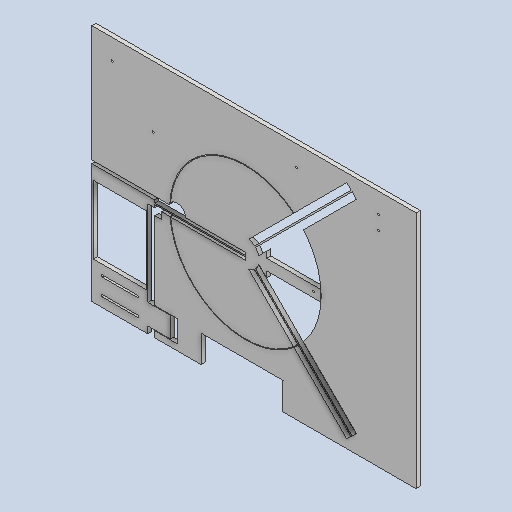
# Autodesk Inventor part: Wheel1
Saved by Autodesk Inventor 2023 (Build 270158000, 158)
## iProperties
Created: 2023-05-10
Part Number: Wheel1
Material: Generic
Document SubType Name: Modeling
Designer: Nathann
Density: 1 g/cm^3
Appearance: Default
Author: Nathann
Autodesk Inventor part; units mm, degrees
ref_plane "YZ Plane" through (0, 0, 0) normal (1, 0, 0) x (0, 1, 0)
ref_plane "XZ Plane" through (0, 0, 0) normal (0, 1, 0) x (-1, 0, 0)
ref_plane "XY Plane" through (0, 0, 0) normal (0, 0, 1) x (1, 0, 0)
sketch "Sketch1" plane through (0, 0, 0) normal (0, 0, 1) x (1, 0, 0)
  line L0 (0, 0) -> (-400, 0)
  line L1 (-400, 0) -> (-400, 350)
  line L2 (-400, 350) -> (0, 350)
  line L3 (0, 350) -> (0, 0)
  circle A0 centre (-175, 175) radius 110
  circle A1 centre (-175, 175) radius 20
  line L4 (-160.8579, 160.8579) -> (0, 0)
  line L5 (0, 350) -> (-160.8579, 189.1421)
  line L6 (-169.8236, 194.3185) -> (-26.5076, 337.6346)
  line L7 (-26.5076, 337.6346) -> (-12.3654, 323.4924)
  line L8 (-12.3654, 323.4924) -> (-155.6815, 180.1764)
  line L9 (-155.6815, 169.8236) -> (-12.1198, 26.262)
  line L10 (-169.8236, 155.6815) -> (-26.7532, 12.6111)
  line L11 (-26.7532, 12.6111) -> (-12.1198, 26.262)
  line L12 (-160.1684, 188.4173) -> (-18.7294, 329.8564)
  line L13 (-20.1436, 331.2706) -> (-161.5827, 189.8316)
  line L14 (-160.1684, 161.5827) -> (-18.7048, 20.1191)
  line L15 (-20.1682, 18.754) -> (-161.5827, 160.1684)
  circle A2 centre (-175, 175) radius 111
  line L16 (-400, 0) -> (-317.8714, 0)
  line L17 (-317.8714, 0) -> (-317.8714, 55)
  line L18 (-317.8714, 55) -> (-400, 55)
  line L19 (-400, 55) -> (-400, 0)
  line L20 (-317.8714, 0) -> (-307.8714, 0)
  line L21 (-307.8714, 0) -> (-307.8714, 155)
  line L22 (-317.8714, 155) -> (-317.8714, 0)
  line L23 (-317.8714, 55) -> (-320.1214, 55)
  line L24 (-320.1214, 55) -> (-320.1214, 155)
  line L25 (-320.1214, 155) -> (-317.8714, 155)
  line L26 (-317.8714, 155) -> (-317.8714, 55)
  line L27 (-400, 55) -> (-397.75, 55)
  line L28 (-397.75, 55) -> (-397.75, 155)
  line L29 (-397.75, 155) -> (-400, 155)
  line L30 (-400, 155) -> (-400, 55)
  line L31 (-400, 155) -> (-307.8714, 155)
  line L32 (-307.8714, 155) -> (-307.8714, 175)
  line L33 (-307.8714, 175) -> (-400, 175)
  line L34 (-400, 175) -> (-400, 155)
  line L35 (-175, 175) -> (-307.8714, 175)
  line L36 (-307.8714, 175) -> (-307.8714, 171)
  line L37 (-307.8714, 171) -> (-175, 171)
  line L38 (-175, 171) -> (-175, 175)
  line L39 (-307.8714, 169) -> (-175, 169)
  line L40 (-175, 169) -> (-175, 165)
  line L41 (-175, 165) -> (-307.8714, 165)
  line L42 (-307.8714, 165) -> (-307.8714, 169)
  line L43 (-317.8714, 155) -> (-297.8714, 155)
  line L44 (-297.8714, 155) -> (-297.8714, 165)
  line L45 (-297.8714, 165) -> (-317.8714, 165)
  line L46 (-317.8714, 165) -> (-317.8714, 155)
  line L47 (-400, 175) -> (-285.6082, 175)
  line L48 (-285.6082, 175) -> (-285.6082, 179.6746)
  line L49 (-285.6082, 179.6746) -> (-400, 179.6746)
  line L50 (-400, 179.6746) -> (-400, 175)
  line L51 (-317.8714, 40) -> (-285, 40)
  line L52 (-285, 40) -> (-285, 10)
  line L53 (-285, 10) -> (-317.8714, 10)
  line L54 (-317.8714, 10) -> (-317.8714, 40)
  line L55 (-307.8714, 53.2478) -> (-275, 53.2478)
  line L56 (-275, 53.2478) -> (-275, 41)
  line L57 (-275, 41) -> (-307.8714, 41)
  line L58 (-307.8714, 41) -> (-307.8714, 53.2478)
  line L59 (-275, 53.2478) -> (-257.3747, 53.2478)
  line L60 (-257.3747, 53.2478) -> (-257.3747, 0)
  line L61 (-257.3747, 0) -> (-275, 0)
  line L62 (-275, 0) -> (-275, 53.2478)
  line L63 (-275, 0) -> (-307.8714, 0)
  line L64 (-307.8714, 0) -> (-307.8714, 9)
  line L65 (-307.8714, 9) -> (-275, 9)
  line L66 (-275, 9) -> (-275, 0)
  point P0 (-19.4365, 330.5635)
  point P1 (-19.4365, 19.4365)
  point P2 (-89.7592, 246.0986)
  point P3 (-89.7592, 103.9014)
  point P4 (-90.4693, 104.6114)
  point P5 (-90.4693, 245.3886)
  point P6 (-104.6114, 259.5307)
  point P7 (-104.6114, 90.4693)
  point P8 (-103.9014, 89.7592)
  point P9 (-103.9014, 260.2408)
  point P10 (-317.8714, 27.5)
  point P11 (-285.5486, 165)
  point P12 (-284.5445, 165)
  point P13 (-317.8714, 0)
  point P14 (-285, 175)
  point P15 (-286, 175)
  point P16 (-285.8377, 169)
  point P17 (-194.0788, 169)
  point P18 (-192.3205, 165)
  point P19 (-97.9286, 96.5144)
  point P20 (-97.2214, 95.8072)
  point P21 (-284.8362, 169)
  point P22 (-96.5144, 97.9286)
  point P23 (-96.5144, 252.0714)
  point P24 (-97.9286, 253.4856)
  point P25 (-97.2214, 254.1928)
  point P26 (-95.8072, 252.7786)
  point P27 (-95.8072, 97.2214)
  point P28 (-285.9015, 179.6746)
  point P29 (-312.8714, 0)
  dimension "d7" = 40
  dimension "d0" = 350
  dimension "d1" = 400
  dimension "d4" = 175
  dimension "d5" = 175
  dimension "d6" = 220
  dimension "d8" = 10
  dimension "d9" = 10
  dimension "d10" = 10
  dimension "d11" = 10
  dimension "d12" = 1
  dimension "d13" = 1
  dimension "d14" = 1
  dimension "d15" = 1
  dimension "d16" = 200
  dimension "d17" = 200
  dimension "d18" = 222
  dimension "d19" = 100
  dimension "d20" = 2.25
  dimension "d21" = 2.25
  dimension "d22" = 10
  dimension "d24" = 20
  dimension "d25" = 0
  dimension "d26" = 6
  dimension "d27" = 4
  dimension "d28" = 4
  dimension "d29" = 20
  dimension "d30" = 0
  dimension "d31" = 1
  dimension "d32" = 1
  dimension "d33" = 10
  dimension "d34" = 30
  dimension "d35" = 10
  constraints: 134 end point, 33 parallel, 16 perpendicular, 15 point on line, 14 horizontal, 4 midpoint, 2 centre point, 2 coincident, 12 other
  measures "d0" distance of L2.end L0.start
  measures "d1" distance of L0.start L0.end
  measures "d4" distance from line of L3 A0.centre
  measures "d5" distance from line of L0 A0.centre
  measures "d6" diameter of A0
  measures "d8" distance between parallel lines of L6 L5
  measures "d9" distance between parallel lines of L8 L5
  measures "d10" distance between parallel lines of L9 L4
  measures "d11" distance between parallel lines of L4 L10
  measures "d12" distance between parallel lines of L13 L5
  measures "d13" distance between parallel lines of L12 L5
  measures "d14" distance between parallel lines of L14 L4
  measures "d15" distance between parallel lines of L15 L4
  measures "d16" distance of point (-19.437, 330.563) L5.end
  measures "d17" distance of point (-19.437, 19.437) L4.start
  measures "d18" diameter of A2
  measures "d19" distance between parallel lines of L18 L31
  measures "d20" distance between parallel lines of L24 L26
  measures "d21" distance between parallel lines of L1 L28
  measures "d22" distance from line of point (-317.871, 27.5) L21
  measures "d24" distance between parallel lines of L31 L33
  measures "d25" distance from line of L33 point (-175, 175)
  measures "d26" distance from line of L39 A0.centre
  measures "d27" distance between parallel lines of L41 L39
  measures "d28" distance between parallel lines of L35 L37
  measures "d29" distance between parallel lines of L46 L44
  measures "d30" distance from line of point (-175, 175) L35
  measures "d31" distance between parallel lines of L65 L53
  measures "d32" distance between parallel lines of L51 L57
  measures "d33" distance between parallel lines of L62 L52
  measures "d34" distance of L51.end L52.end
  measures "d35" distance from line of point (-312.871, 0) L53
extrude "Extrusion1" add sketch "Sketch1" along normal blind 6 contours L4 L11 L9 A2 L8 L7 L5 L3 | L0 L60 L59 L55 L21 L43 L44 L41 A2 L10 L11 L4 | L0 L62 L56 L59 L60 | L5 L7 L6 A2 L49 L1 L2 | L11 L15 A2 L4 | L4 A2 L14 L11 | L0 L21 L65 L62 | L7 L12 A2 L5 | L5 A2 L13 L7 | A2 L15 A0 L4 | L4 A0 L14 A2 | L56 L57 L21 L55 | A2 L12 A0 L5 | L5 A0 L13 A2 | L4 A1 L14 A0 | A0 L15 A1 L4 | L0 L1 L18 L17 | L33 L32 L45 L46 L25 L31 L29 L1 | L5 A1 L13 A0 | A0 L12 A1 L5 | A1 L41 L40 L39 L37 L38 L35 | L17 L51 L21 L53 | L21 L51 L52 L53 | L29 L28 L18 L1 | A0 L41 A1 L10 | L9 A1 L8 A0 | L22 L18 L24 L25 | L37 A2 L39 L32 | L6 A1 L35 A0 | L37 A0 L39 A2 | L37 A1 L39 A0
sketch "Sketch2" plane through (0, 0, 0) normal (0, 0, -1) x (-1, 0, 0)
  circle A0 centre (75, 175) radius 1.5
  arc A1 (89.7592, 246.0986) -> (89.7592, 103.9014) centre (175, 175) ccw projected
  circle A2 centre (275.0738, 175.0894) radius 1.5 projected
  circle A3 centre (275.0738, 175.0894) radius 12.5
  line L0 (262.7011, 173.3102) -> (287.4465, 173.3102)
  point P0 (0, 0)
  dimension "d36" = 100
  dimension "d37" = 0
  dimension "d38" = 3
  dimension "d41" = 25
  constraints: 2 centre point, 2 end point, 2 point on circle, 1 coincident, 1 horizontal
  measures "d36" distance of A1.centre A0.centre
  measures "d37" vertical distance of A1.centre A0.centre
  measures "d38" diameter of A0
  measures "d41" diameter of A3
extrude "Extrusion2" cut sketch "Sketch2" against normal blind 6 contours A0 | A2 | A3 L0 picked at (283.793, 176.058)
sketch "Sketch3" plane through (0, 0, 0) normal (0, 0, -1) x (-1, 0, 0)
  line L0 (307.8714, 0) -> (0, 0) projected
  line L1 (240, 0) -> (120, 0)
  line L2 (120, 0) -> (120, 40)
  line L3 (120, 40) -> (240, 40)
  line L4 (240, 40) -> (240, 0)
  line L5 (0, 0) -> (0, 350) projected
  point P0 (120, 0)
  dimension "d42" = 40
  dimension "d43" = 120
  dimension "d44" = 120
  constraints: 8 end point, 2 parallel, 1 horizontal, 1 perpendicular, 1 point on line
  measures "d42" distance of L1.end L2.end
  measures "d43" distance of L2.end L3.end
  measures "d44" distance between parallel lines of L5 L2
extrude "Extrusion3" cut sketch "Sketch3" against normal blind 6
sketch "Sketch4" plane through (0, 0, 0) normal (0, 0, -1) x (-1, 0, 0)
  circle A0 centre (370, 320) radius 1.5
  circle A1 centre (100, 320) radius 1.5
  circle A2 centre (310, 260) radius 1.5
  line L0 (0, 350) -> (400, 350) projected
  line L1 (400, 350) -> (400, 179.6746) projected
  line L2 (0, 0) -> (0, 350) projected
  dimension "d47" = 3
  dimension "d48" = 30
  dimension "d49" = 30
  dimension "d50" = 90
  dimension "d51" = 90
  dimension "d52" = 3
  dimension "d53" = 3
  dimension "d54" = 100
  dimension "d55" = 30
  constraints: 3 centre point
  measures "d47" diameter of A0
  measures "d48" distance from line of L0 A0.centre
  measures "d49" distance from line of L1 A0.centre
  measures "d50" distance from line of L0 A2.centre
  measures "d51" distance from line of A2.centre L1
  measures "d52" diameter of A2
  measures "d53" diameter of A1
  measures "d54" distance from line of L2 A1.centre
  measures "d55" distance from line of L0 A1.centre
extrude "Extrusion4" cut sketch "Sketch4" against normal blind 6
sketch "Sketch5" plane through (0, 0, 0) normal (0, 0, -1) x (-1, 0, 0)
  line L0 (65.2913, 167) -> (143.7852, 167)
  line L1 (65.2913, 183) -> (143.7852, 183)
  circle A0 centre (75, 175) radius 1.5 projected
  circle A1 centre (100, 320) radius 1.5 projected
  circle A2 centre (310, 260) radius 1.5 projected
  circle A3 centre (370, 320) radius 1.5 projected
  line L2 (240, 40) -> (240, 0) projected
  line L3 (307.8714, 0) -> (240, 0) projected
  line L4 (307.8714, 9) -> (307.8714, 0) projected
  line L5 (275, 9) -> (307.8714, 9) projected
  line L6 (275, 41) -> (275, 9) projected
  line L7 (307.8714, 41) -> (275, 41) projected
  line L8 (307.8714, 155) -> (307.8714, 41) projected
  line L9 (297.8714, 155) -> (307.8714, 155) projected
  line L10 (297.8714, 165) -> (297.8714, 155) projected
  line L11 (285.5486, 165) -> (297.8714, 165) projected
  arc A4 (103.9014, 89.7592) -> (285.5486, 165) centre (175, 175) ccw projected
  line L12 (26.7532, 12.6111) -> (103.9014, 89.7592) projected
  line L13 (20.1682, 18.754) -> (26.7532, 12.6111) projected
  line L14 (161.5827, 160.1684) -> (20.1682, 18.754) projected
  arc A5 (161.5827, 160.1684) -> (169.8236, 155.6815) centre (175, 175) ccw projected
  line L15 (104.6114, 90.4693) -> (169.8236, 155.6815) projected
  arc A6 (104.6114, 90.4693) -> (284.5445, 165) centre (175, 175) ccw projected
  line L16 (175, 165) -> (284.5445, 165) projected
  line L17 (175, 169) -> (175, 165) projected
  line L18 (307.8714, 169) -> (175, 169) projected
  line L19 (307.8714, 165) -> (307.8714, 169) projected
  line L20 (317.8714, 165) -> (307.8714, 165) projected
  line L21 (317.8714, 40) -> (317.8714, 165) projected
  line L22 (285, 40) -> (317.8714, 40) projected
  line L23 (285, 10) -> (285, 40) projected
  line L24 (317.8714, 10) -> (285, 10) projected
  line L25 (317.8714, 0) -> (317.8714, 10) projected
  line L26 (400, 0) -> (317.8714, 0) projected
  line L27 (400, 175) -> (400, 0) projected
  line L28 (307.8714, 175) -> (400, 175) projected
  line L29 (307.8714, 171) -> (307.8714, 175) projected
  line L30 (175, 171) -> (307.8714, 171) projected
  line L31 (175, 175) -> (175, 171) projected
  line L32 (262.5741, 175) -> (175, 175) projected
  arc A7 (284.7044, 183.0581) -> (262.5741, 175) centre (275.0738, 175.0894) ccw projected
  arc A8 (284.7044, 183.0581) -> (104.6114, 259.5307) centre (175, 175) ccw projected
  line L33 (169.8236, 194.3185) -> (104.6114, 259.5307) projected
  arc A9 (169.8236, 194.3185) -> (161.5827, 189.8316) centre (175, 175) ccw projected
  line L34 (20.1436, 331.2706) -> (161.5827, 189.8316) projected
  line L35 (26.5076, 337.6346) -> (20.1436, 331.2706) projected
  line L36 (103.9014, 260.2408) -> (26.5076, 337.6346) projected
  arc A10 (285.81, 181.4913) -> (103.9014, 260.2408) centre (175, 175) ccw projected
  arc A11 (286.7025, 179.6746) -> (285.81, 181.4913) centre (275.0738, 175.0894) ccw projected
  line L37 (400, 179.6746) -> (286.7025, 179.6746) projected
  line L38 (400, 350) -> (400, 179.6746) projected
  line L39 (0, 350) -> (400, 350) projected
  line L40 (0, 0) -> (0, 350) projected
  line L41 (120, 0) -> (0, 0) projected
  line L42 (120, 0) -> (120, 40) projected
  line L43 (120, 40) -> (240, 40) projected
  line L44 (160.1684, 188.4173) -> (18.7294, 329.8564) projected
  arc A12 (160.1684, 188.4173) -> (155.6815, 180.1764) centre (175, 175) ccw projected
  line L45 (90.4693, 245.3886) -> (155.6815, 180.1764) projected
  arc A13 (90.4693, 245.3886) -> (90.4693, 104.6114) centre (175, 175) ccw projected
  line L46 (155.6815, 169.8236) -> (90.4693, 104.6114) projected
  arc A14 (155.6815, 169.8236) -> (160.1684, 161.5827) centre (175, 175) ccw projected
  line L47 (18.7048, 20.1191) -> (160.1684, 161.5827) projected
  line L48 (12.1198, 26.262) -> (18.7048, 20.1191) projected
  line L49 (89.7592, 103.9014) -> (12.1198, 26.262) projected
  arc A15 (89.7592, 246.0986) -> (89.7592, 103.9014) centre (175, 175) ccw projected
  line L50 (12.3654, 323.4924) -> (89.7592, 246.0986) projected
  line L51 (18.7294, 329.8564) -> (12.3654, 323.4924) projected
  line L52 (397.75, 155) -> (320.1214, 155) projected
  line L53 (397.75, 55) -> (397.75, 155) projected
  line L54 (320.1214, 55) -> (397.75, 55) projected
  line L55 (320.1214, 155) -> (320.1214, 55) projected
  circle A16 centre (75, 175) radius 1.5 projected
  line L56 (143.7852, 167) -> (143.7852, 157.9273)
  line L57 (143.7852, 183) -> (143.7852, 192.0727)
  dimension "d61" = 8
  dimension "d62" = 8
  constraints: 8 end point, 2 horizontal, 2 perpendicular, 2 point on circle, 2 point on line
  measures "d61" distance from line of L1 A0.centre
  measures "d62" distance from line of A0.centre L0
extrude "Extrusion5" cut sketch "Sketch5" against normal blind 10 contours L0 L56 L46 A13 | A13 L45 L57 L1
sketch "Sketch6" plane through (0, 0, 6) normal (0, 0, 1) x (1, 0, 0)
  circle A0 centre (-385, 15) radius 1.5
  circle A1 centre (-385, 40) radius 1.5
  circle A2 centre (-332.8714, 40) radius 1.5
  circle A3 centre (-332.8714, 15) radius 1.5
  line L0 (-400, 0) -> (-317.8714, 0) projected
  line L1 (-400, 175) -> (-400, 0) projected
  line L2 (-317.8714, 0) -> (-317.8714, 10) projected
  line L3 (-317.8714, 40) -> (-317.8714, 165) projected
  line L4 (-320.1214, 55) -> (-397.75, 55) projected
  line L5 (-385, 41.5) -> (-332.8714, 41.5)
  line L6 (-332.8714, 38.5) -> (-385, 38.5)
  line L7 (-385, 16.5) -> (-332.8714, 16.5)
  line L8 (-332.8714, 13.5) -> (-385, 13.5)
  point P0 (0, 0)
  dimension "d65" = 15
  dimension "d66" = 15
  dimension "d67" = 15
  dimension "d68" = 15
  dimension "d69" = 15
  dimension "d70" = 15
  dimension "d71" = 15
  dimension "d72" = 15
  dimension "d73" = 3
  dimension "d74" = 3
  dimension "d75" = 3
  dimension "d76" = 3
  dimension "d77" = 52.1286
  dimension "d80" = 25
  constraints: 8 end point, 8 point on circle, 4 centre point, 4 tangent
  measures "d65" distance from line of L0 A0.centre
  measures "d66" distance from line of L1 A0.centre
  measures "d67" distance from line of L0 A3.centre
  measures "d68" distance from line of L2 A3.centre
  measures "d69" distance from line of L3 A2.centre
  measures "d70" distance from line of L4 A2.centre
  measures "d71" distance from line of L4 A1.centre
  measures "d72" distance from line of L1 A1.centre
  measures "d73" diameter of A1
  measures "d74" diameter of A0
  measures "d75" diameter of A3
  measures "d76" diameter of A2
  measures "d77" distance of A2.centre A1.centre
  measures "d80" distance of A0.centre A1.centre
extrude "Extrusion6" cut sketch "Sketch6" against normal blind 10
sketch "Sketch7" plane through (0, 0, 6) normal (0, 0, 1) x (1, 0, 0)
  line L0 (0, 0) -> (0, 350) projected
  line L1 (0, 0) -> (75, 0)
  line L2 (75, 0) -> (75, 350)
  line L3 (75, 350) -> (0, 350)
  line L4 (0, 350) -> (0, 0)
  line L5 (-400, 350) -> (-400, 179.6746) projected
  dimension "d81" = 475
  constraints: 8 end point, 2 parallel, 1 horizontal, 1 perpendicular
  measures "d81" distance between parallel lines of L2 L5
extrude "Extrusion7" add sketch "Sketch7" against normal blind 6
sketch "Sketch8" plane through (0, 0, 6) normal (0, 0, 1) x (1, 0, 0)
  line L0 (35, 298.5) -> (7.1582, 298.5001) projected
  line L1 (7.1582, 301.5001) -> (35, 301.5) projected
  line L2 (7.275, 321.4955) -> (35.1179, 321.4954) projected
  line L3 (35, 318.5) -> (7.1745, 318.5001) projected
  circle A0 centre (20, 300) radius 1.5
  circle A1 centre (20, 320) radius 1.5
  point P0 (0, 0)
  point P1 (20.1179, 321.4954)
  point P2 (19.8821, 321.4954)
  dimension "d84" = 3
  dimension "d85" = 3
  dimension "d86" = 15
  dimension "d87" = 15
  constraints: 2 centre point, 2 tangent
  measures "d84" diameter of A0
  measures "d85" diameter of A1
  measures "d86" horizontal distance of L3.start A1.centre
  measures "d87" horizontal distance of L0.start A0.centre
extrude "Extrusion8" cut sketch "Sketch8" against normal blind 6 contours L2 A1 | A0 picked at (20.4394, 320.3505)
equation "\"d4\" = d5"
equation "\"d5\" = 0.5 * d0"
equation "\"d13\" = d12"
equation "\"d15\" = d14"
equation "\"d16\" = BladeLengthRCC"
equation "\"d17\" = d16"
equation "\"d19\" = bladeLengthZeroConverter"
equation "\"d20\" = bladeThicknessZeroConverter"
equation "\"d21\" = bladeThicknessZeroConverter"
equation "\"d27\" = d28"
equation "\"d2\" = thicknessWheelPlate"
equation "\"d39\" = thicknessWheelPlate"
equation "\"d45\" = thicknessWheelPlate"
equation "\"d56\" = thicknessWheelPlate"
equation "\"d68\" = d66"
equation "\"d69\" = d68"
equation "\"d70\" = d67"
equation "\"d71\" = d70"
equation "\"d72\" = d71"
equation "\"d73\" = d76"
equation "\"d74\" = d75"
equation "\"d76\" = d75"
equation "\"bladeThicknessTablePushing\" = 1"
equation "\"bladeThicknessTable\" = 1"
equation "\"bladeThicknessForceConverter\" = 2"
equation "\"bladeThicknessWheelAnchor\" = 1"
equation "\"BladeThicknessRCC\" = 1"
equation "\"bladeThicknessZeroConverter\" = 2.25"
equation "\"rangeXProbeMax\" = 1"
equation "\"rangeXProbeMin\" = -1"
equation "\"BladeLengthRCC\" = 200"
equation "\"bladeLengthZeroConverter\" = 100"
equation "\"safetyPlay\" = 0.1"
equation "\"OffsetMotorSpring\" = -1"
equation "\"thicknessWheelPlate\" = 6"
equation "\"thicknessConverterPlate\" = 6"
body "Solid1"
